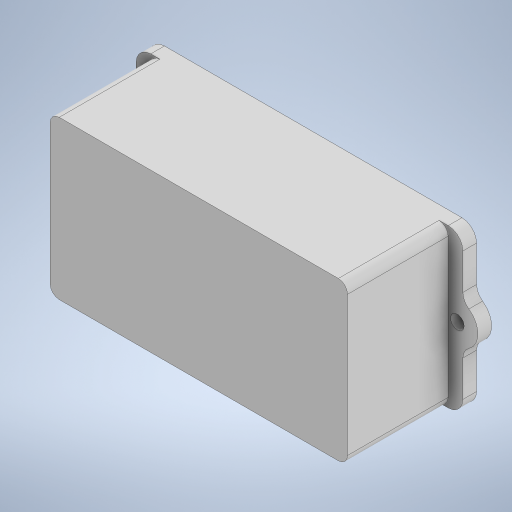
# Autodesk Inventor part: верхняя часть держателя аккумулятора
Saved by Autodesk Inventor 2023.1 (Build 271208000, 208)
## iProperties
Created: 2023-02-23
Part Number: верхняя часть держателя аккумулятора
Material: Типовые
Document SubType Name: Modeling
Designer: User
Density: 1 g/cm^3
Appearance: По умолчанию
Author: User
Autodesk Inventor part; units mm, degrees
ref_plane "YZ Plane" through (0, 0, 0) normal (1, 0, 0) x (0, 1, 0)
ref_plane "XZ Plane" through (0, 0, 0) normal (0, 1, 0) x (-1, 0, 0)
ref_plane "XY Plane" through (0, 0, 0) normal (0, 0, 1) x (1, 0, 0)
sketch "Эскиз1" plane through (0, 0, 0) normal (0, 0, 1) x (1, 0, 0)
  arc A0 (32.5, -17.25) -> (35.7, -14.05) centre (32.5, -14.05) ccw
  line L0 (35.7, -14.05) -> (35.7, -6.2137)
  arc A1 (37.02, -3.7282) -> (35.7, -6.2137) centre (38.7, -6.2137) ccw
  arc A2 (37.02, -3.7282) -> (37.02, 3.7282) centre (34.5, 0) ccw
  arc A3 (35.7, 6.2137) -> (37.02, 3.7282) centre (38.7, 6.2137) ccw
  line L1 (35.7, 6.2137) -> (35.7, 14.05)
  arc A4 (35.7, 14.05) -> (32.5, 17.25) centre (32.5, 14.05) ccw
  line L2 (32.5, 17.25) -> (-32.5, 17.25)
  arc A5 (-32.5, 17.25) -> (-35.7, 14.05) centre (-32.5, 14.05) ccw
  line L3 (-35.7, 14.05) -> (-35.7, 6.2137)
  arc A6 (-37.02, 3.7282) -> (-35.7, 6.2137) centre (-38.7, 6.2137) ccw
  arc A7 (-37.02, 3.7282) -> (-37.02, -3.7282) centre (-34.5, 0) ccw
  arc A8 (-35.7, -6.2137) -> (-37.02, -3.7282) centre (-38.7, -6.2137) ccw
  line L4 (-35.7, -6.2137) -> (-35.7, -14.05)
  arc A9 (-35.7, -14.05) -> (-32.5, -17.25) centre (-32.5, -14.05) ccw
  line L5 (-32.5, -17.25) -> (32.5, -17.25)
  line L6 (30.5, -15) -> (-30.5, -15)
  line L7 (-30.5, -15) -> (-30.5, 15)
  line L8 (-30.5, 15) -> (30.5, 15)
  line L9 (30.5, 15) -> (30.5, -15)
  circle A10 centre (-34.5, 0) radius 1.5
  circle A11 centre (34.5, 0) radius 1.5
  point P0 (0, 0)
  point P1 (-32.5, -17.25)
  point P2 (32.5, -17.25)
  point P3 (32.5, 17.25)
  point P4 (-35.7, 14.05)
  point P5 (-37.02, 3.7282)
  point P6 (-37.02, -3.7282)
  constraints: 20 end point, 20 point on circle, 12 centre point
extrude "Выдавливание1" add sketch "Эскиз1" along normal blind 3
sketch "Эскиз2" plane through (0, 0, 3) normal (0, 0, 1) x (1, 0, 0)
  line L0 (32.5, 17.25) -> (-32.5, 17.25) projected
  line L1 (-32.5, -17.25) -> (32.5, -17.25) projected
  line L2 (-32.5, 17.25) -> (32.5, 17.25)
  line L3 (32.5, 17.25) -> (32.5, -17.25)
  line L4 (32.5, -17.25) -> (-32.5, -17.25)
  line L5 (-32.5, -17.25) -> (-32.5, 17.25)
  line L6 (-30.5, 15) -> (30.5, 15) projected
  line L7 (-30.5, -15) -> (-30.5, 15) projected
  line L8 (30.5, -15) -> (-30.5, -15) projected
  line L9 (30.5, 15) -> (30.5, -15) projected
  point P0 (0, 0)
  constraints: 8 end point, 2 parallel, 1 horizontal, 1 perpendicular
extrude "Выдавливание2" add sketch "Эскиз2" along normal blind 20
fillet "Сопряжение1" radius 2 4 edges at (-32.5, -17.25, 13) (32.5, -17.25, 13) (32.5, 17.25, 13) (-32.5, 17.25, 13)
sketch "Эскиз3" plane through (0, 0, 23) normal (0, 0, 1) x (1, 0, 0)
  line L0 (30.5, 17.25) -> (-30.5, 17.25) projected
  arc A0 (-30.5, 17.25) -> (-32.5, 15.25) centre (-30.5, 15.25) ccw projected
  line L1 (-32.5, 15.25) -> (-32.5, -15.25) projected
  arc A1 (-32.5, -15.25) -> (-30.5, -17.25) centre (-30.5, -15.25) ccw projected
  line L2 (-30.5, -17.25) -> (30.5, -17.25) projected
  arc A2 (30.5, -17.25) -> (32.5, -15.25) centre (30.5, -15.25) ccw projected
  line L3 (32.5, -15.25) -> (32.5, 15.25) projected
  arc A3 (32.5, 15.25) -> (30.5, 17.25) centre (30.5, 15.25) ccw projected
  line L4 (30.5, 17.25) -> (-30.5, 17.25) projected
  line L5 (-30.5, 15) -> (30.5, 15) projected
  line L6 (30.5, 15) -> (30.5, -15) projected
  line L7 (30.5, -15) -> (-30.5, -15) projected
  line L8 (-30.5, -15) -> (-30.5, 15) projected
  point P0 (0, 0)
extrude "Выдавливание3" add sketch "Эскиз3" along normal blind 2 contours A3 L3 A2 L2 A1 L1 A0 L0 | L5 L6 L7 L8
sketch "Эскиз4" plane through (-32.5, -17.25, 0) normal (0, -1, 0) x (1, 0, 0)
  line L0 (0.3457, 22.1232) -> (67.4397, 22.1232) construction
  line L1 (67.4397, 22.1232) -> (67.4397, 17.9316) construction
  line L2 (67.4397, 17.9316) -> (0.3457, 17.9316) construction
  line L3 (0.3457, 17.9316) -> (0.3457, 22.1232) construction
  line L4 (7.2699, 17.9367) -> (6.3706, 17.9367)
  spline S0 degree 2 poles (6.3706, 17.9367) (6.0759, 17.9367) (6.0759, 18.2364) knots 0 0 0 1 1 1
  spline S1 degree 2 poles (6.0759, 18.2364) (6.0759, 18.5362) (6.3706, 18.5362) knots 0 0 0 1 1 1
  line L5 (6.3706, 18.5362) -> (7.2699, 18.5362)
  line L6 (7.2699, 18.5362) -> (7.2699, 19.1357)
  spline S2 degree 2 poles (7.2699, 19.1357) (7.2699, 19.3805) (6.9152, 19.7302) (6.6704, 19.7302) knots 0 0 0 1 2 2 2
  line L7 (6.6704, 19.7302) -> (5.1766, 19.7302)
  spline S3 degree 2 poles (5.1766, 19.7302) (4.8769, 19.7302) (4.8769, 20.0299) knots 0 0 0 1 1 1
  spline S4 degree 2 poles (4.8769, 20.0299) (4.8769, 20.3297) (5.1766, 20.3297) knots 0 0 0 1 1 1
  line L8 (5.1766, 20.3297) -> (6.6704, 20.3297)
  spline S5 degree 2 poles (6.6704, 20.3297) (7.17, 20.3297) (7.8694, 19.6303) (7.8694, 19.1357) knots 0 0 0 1 2 2 2
  line L9 (7.8694, 19.1357) -> (7.8694, 17.3372)
  spline S6 degree 2 poles (7.8694, 17.3372) (7.8694, 16.8426) (7.17, 16.1432) (6.6704, 16.1432) knots 0 0 0 1 2 2 2
  line L10 (6.6704, 16.1432) -> (5.1766, 16.1432)
  spline S7 degree 2 poles (5.1766, 16.1432) (4.8769, 16.1432) (4.8769, 16.4429) knots 0 0 0 1 1 1
  spline S8 degree 2 poles (4.8769, 16.4429) (4.8769, 16.7427) (5.1766, 16.7427) knots 0 0 0 1 1 1
  line L11 (5.1766, 16.7427) -> (6.6704, 16.7427)
  spline S9 degree 2 poles (6.6704, 16.7427) (6.9152, 16.7427) (7.2699, 17.0974) (7.2699, 17.3422) knots 0 0 0 1 2 2 2
  line L12 (7.2699, 17.3422) -> (7.2699, 17.9367)
  line L13 (10.8619, 19.7302) -> (9.6679, 19.7302)
  line L14 (9.6679, 19.7302) -> (9.6679, 16.4429)
  spline S10 degree 2 poles (9.6679, 16.4429) (9.6679, 16.1432) (9.3681, 16.1432) knots 0 0 0 1 1 1
  spline S11 degree 2 poles (9.3681, 16.1432) (9.0684, 16.1432) (9.0684, 16.4429) knots 0 0 0 1 1 1
  line L15 (9.0684, 16.4429) -> (9.0684, 20.0299)
  spline S12 degree 2 poles (9.0684, 20.0299) (9.0684, 20.3297) (9.3681, 20.3297) knots 0 0 0 1 1 1
  line L16 (9.3681, 20.3297) -> (12.0609, 20.3297)
  spline S13 degree 2 poles (12.0609, 20.3297) (12.5555, 20.3297) (13.2549, 19.6303) (13.2549, 19.1357) knots 0 0 0 1 2 2 2
  line L17 (13.2549, 19.1357) -> (13.2549, 16.4429)
  spline S14 degree 2 poles (13.2549, 16.4429) (13.2549, 16.1432) (12.9551, 16.1432) knots 0 0 0 1 1 1
  spline S15 degree 2 poles (12.9551, 16.1432) (12.6554, 16.1432) (12.6554, 16.4429) knots 0 0 0 1 1 1
  line L18 (12.6554, 16.4429) -> (12.6554, 19.1307)
  spline S16 degree 2 poles (12.6554, 19.1307) (12.6554, 19.3755) (12.3057, 19.7302) (12.0609, 19.7302) knots 0 0 0 1 2 2 2
  line L19 (12.0609, 19.7302) -> (11.4614, 19.7302)
  line L20 (11.4614, 19.7302) -> (11.4614, 16.4429)
  spline S17 degree 2 poles (11.4614, 16.4429) (11.4614, 16.1432) (11.1616, 16.1432) knots 0 0 0 1 1 1
  spline S18 degree 2 poles (11.1616, 16.1432) (10.8619, 16.1432) (10.8619, 16.4429) knots 0 0 0 1 1 1
  line L21 (10.8619, 16.4429) -> (10.8619, 19.7302)
  spline S19 degree 2 poles (17.4414, 17.4571) (17.4414, 16.9075) (16.672, 16.1432) (16.1275, 16.1432) knots 0 0 0 1 2 2 2
  line L22 (16.1275, 16.1432) -> (15.7678, 16.1432)
  spline S20 degree 2 poles (15.7678, 16.1432) (15.2282, 16.1432) (14.4539, 16.9125) (14.4539, 17.4571) knots 0 0 0 1 2 2 2
  line L23 (14.4539, 17.4571) -> (14.4539, 19.0158)
  spline S21 degree 2 poles (14.4539, 19.0158) (14.4539, 19.5603) (15.2282, 20.3297) (15.7678, 20.3297) knots 0 0 0 1 2 2 2
  line L24 (15.7678, 20.3297) -> (16.1275, 20.3297)
  spline S22 degree 2 poles (16.1275, 20.3297) (16.672, 20.3297) (17.4414, 19.5603) (17.4414, 19.0158) knots 0 0 0 1 2 2 2
  line L25 (17.4414, 19.0158) -> (17.4414, 17.4571)
  line L26 (16.8419, 17.4621) -> (16.8419, 19.0108)
  spline S23 degree 2 poles (16.8419, 19.0108) (16.8419, 19.3055) (16.4172, 19.7302) (16.1275, 19.7302) knots 0 0 0 1 2 2 2
  line L27 (16.1275, 19.7302) -> (15.7678, 19.7302)
  spline S24 degree 2 poles (15.7678, 19.7302) (15.473, 19.7302) (15.0534, 19.3055) (15.0534, 19.0108) knots 0 0 0 1 2 2 2
  line L28 (15.0534, 19.0108) -> (15.0534, 17.4621)
  spline S25 degree 2 poles (15.0534, 17.4621) (15.0534, 17.1623) (15.473, 16.7427) (15.7678, 16.7427) knots 0 0 0 1 2 2 2
  line L29 (15.7678, 16.7427) -> (16.1275, 16.7427)
  spline S26 degree 2 poles (16.1275, 16.7427) (16.4172, 16.7427) (16.8419, 17.1623) (16.8419, 17.4621) knots 0 0 0 1 2 2 2
  spline S27 degree 2 poles (21.6329, 16.4429) (21.6329, 16.1432) (21.3332, 16.1432) knots 0 0 0 1 1 1
  line L30 (21.3332, 16.1432) -> (19.8394, 16.1432)
  spline S28 degree 2 poles (19.8394, 16.1432) (19.3448, 16.1432) (18.6404, 16.8426) (18.6404, 17.3422) knots 0 0 0 1 2 2 2
  line L31 (18.6404, 17.3422) -> (18.6404, 20.0349)
  spline S29 degree 2 poles (18.6404, 20.0349) (18.6404, 20.3297) (18.9401, 20.3297) knots 0 0 0 1 1 1
  spline S30 degree 2 poles (18.9401, 20.3297) (19.2399, 20.3297) (19.2399, 20.0349) knots 0 0 0 1 1 1
  line L32 (19.2399, 20.0349) -> (19.2399, 17.3422)
  spline S31 degree 2 poles (19.2399, 17.3422) (19.2399, 17.0974) (19.5946, 16.7427) (19.8394, 16.7427) knots 0 0 0 1 2 2 2
  line L33 (19.8394, 16.7427) -> (21.0334, 16.7427)
  line L34 (21.0334, 16.7427) -> (21.0334, 20.0349)
  spline S32 degree 2 poles (21.0334, 20.0349) (21.0334, 20.3297) (21.3332, 20.3297) knots 0 0 0 1 1 1
  spline S33 degree 2 poles (21.3332, 20.3297) (21.6329, 20.3297) (21.6329, 20.0349) knots 0 0 0 1 1 1
  line L35 (21.6329, 20.0349) -> (21.6329, 16.4429)
  line L36 (20.7337, 21.5237) -> (19.5396, 21.5237)
  spline S34 degree 2 poles (19.5396, 21.5237) (19.2399, 21.5237) (19.2399, 21.8234) knots 0 0 0 1 1 1
  spline S35 degree 2 poles (19.2399, 21.8234) (19.2399, 22.1232) (19.5396, 22.1232) knots 0 0 0 1 1 1
  line L37 (19.5396, 22.1232) -> (20.7337, 22.1232)
  spline S36 degree 2 poles (20.7337, 22.1232) (21.0334, 22.1232) (21.0334, 21.8234) knots 0 0 0 1 1 1
  spline S37 degree 2 poles (21.0334, 21.8234) (21.0334, 21.5237) (20.7337, 21.5237) knots 0 0 0 1 1 1
  line L38 (28.5122, 16.1432) -> (27.6179, 16.1432)
  spline S38 degree 2 poles (27.6179, 16.1432) (27.1283, 16.1432) (26.4189, 16.8426) (26.4189, 17.3372) knots 0 0 0 1 2 2 2
  line L39 (26.4189, 17.3372) -> (26.4189, 19.1357)
  spline S39 degree 2 poles (26.4189, 19.1357) (26.4189, 19.6303) (27.1283, 20.3297) (27.6179, 20.3297) knots 0 0 0 1 2 2 2
  line L40 (27.6179, 20.3297) -> (28.5122, 20.3297)
  spline S40 degree 2 poles (28.5122, 20.3297) (28.8119, 20.3297) (28.8119, 20.0299) knots 0 0 0 1 1 1
  spline S41 degree 2 poles (28.8119, 20.0299) (28.8119, 19.7302) (28.5122, 19.7302) knots 0 0 0 1 1 1
  line L41 (28.5122, 19.7302) -> (27.6179, 19.7302)
  spline S42 degree 2 poles (27.6179, 19.7302) (27.3731, 19.7302) (27.0184, 19.3755) (27.0184, 19.1307) knots 0 0 0 1 2 2 2
  line L42 (27.0184, 19.1307) -> (27.0184, 17.3422)
  spline S43 degree 2 poles (27.0184, 17.3422) (27.0184, 17.0974) (27.3731, 16.7427) (27.6179, 16.7427) knots 0 0 0 1 2 2 2
  line L43 (27.6179, 16.7427) -> (28.5122, 16.7427)
  spline S44 degree 2 poles (28.5122, 16.7427) (28.8119, 16.7427) (28.8119, 16.4429) knots 0 0 0 1 1 1
  spline S45 degree 2 poles (28.8119, 16.4429) (28.8119, 16.1432) (28.5122, 16.1432) knots 0 0 0 1 1 1
  line L44 (31.7994, 19.7302) -> (30.6054, 19.7302)
  line L45 (30.6054, 19.7302) -> (30.6054, 16.4429)
  spline S46 degree 2 poles (30.6054, 16.4429) (30.6054, 16.1432) (30.3057, 16.1432) knots 0 0 0 1 1 1
  spline S47 degree 2 poles (30.3057, 16.1432) (30.0059, 16.1432) (30.0059, 16.4429) knots 0 0 0 1 1 1
  line L46 (30.0059, 16.4429) -> (30.0059, 20.0299)
  spline S48 degree 2 poles (30.0059, 20.0299) (30.0059, 20.3297) (30.3057, 20.3297) knots 0 0 0 1 1 1
  line L47 (30.3057, 20.3297) -> (32.9984, 20.3297)
  spline S49 degree 2 poles (32.9984, 20.3297) (33.493, 20.3297) (34.1924, 19.6303) (34.1924, 19.1357) knots 0 0 0 1 2 2 2
  line L48 (34.1924, 19.1357) -> (34.1924, 16.4429)
  spline S50 degree 2 poles (34.1924, 16.4429) (34.1924, 16.1432) (33.8927, 16.1432) knots 0 0 0 1 1 1
  spline S51 degree 2 poles (33.8927, 16.1432) (33.5929, 16.1432) (33.5929, 16.4429) knots 0 0 0 1 1 1
  line L49 (33.5929, 16.4429) -> (33.5929, 19.1307)
  spline S52 degree 2 poles (33.5929, 19.1307) (33.5929, 19.3755) (33.2432, 19.7302) (32.9984, 19.7302) knots 0 0 0 1 2 2 2
  line L50 (32.9984, 19.7302) -> (32.3989, 19.7302)
  line L51 (32.3989, 19.7302) -> (32.3989, 16.4429)
  spline S53 degree 2 poles (32.3989, 16.4429) (32.3989, 16.1432) (32.0992, 16.1432) knots 0 0 0 1 1 1
  spline S54 degree 2 poles (32.0992, 16.1432) (31.7994, 16.1432) (31.7994, 16.4429) knots 0 0 0 1 1 1
  line L52 (31.7994, 16.4429) -> (31.7994, 19.7302)
  spline S55 degree 2 poles (38.3789, 17.4571) (38.3789, 16.9075) (37.6096, 16.1432) (37.065, 16.1432) knots 0 0 0 1 2 2 2
  line L53 (37.065, 16.1432) -> (36.7053, 16.1432)
  spline S56 degree 2 poles (36.7053, 16.1432) (36.1658, 16.1432) (35.3914, 16.9125) (35.3914, 17.4571) knots 0 0 0 1 2 2 2
  line L54 (35.3914, 17.4571) -> (35.3914, 19.0158)
  spline S57 degree 2 poles (35.3914, 19.0158) (35.3914, 19.5603) (36.1658, 20.3297) (36.7053, 20.3297) knots 0 0 0 1 2 2 2
  line L55 (36.7053, 20.3297) -> (37.065, 20.3297)
  spline S58 degree 2 poles (37.065, 20.3297) (37.6096, 20.3297) (38.3789, 19.5603) (38.3789, 19.0158) knots 0 0 0 1 2 2 2
  line L56 (38.3789, 19.0158) -> (38.3789, 17.4571)
  line L57 (37.7794, 17.4621) -> (37.7794, 19.0108)
  spline S59 degree 2 poles (37.7794, 19.0108) (37.7794, 19.3055) (37.3548, 19.7302) (37.065, 19.7302) knots 0 0 0 1 2 2 2
  line L58 (37.065, 19.7302) -> (36.7053, 19.7302)
  spline S60 degree 2 poles (36.7053, 19.7302) (36.4106, 19.7302) (35.9909, 19.3055) (35.9909, 19.0108) knots 0 0 0 1 2 2 2
  line L59 (35.9909, 19.0108) -> (35.9909, 17.4621)
  spline S61 degree 2 poles (35.9909, 17.4621) (35.9909, 17.1623) (36.4106, 16.7427) (36.7053, 16.7427) knots 0 0 0 1 2 2 2
  line L60 (36.7053, 16.7427) -> (37.065, 16.7427)
  spline S62 degree 2 poles (37.065, 16.7427) (37.3548, 16.7427) (37.7794, 17.1623) (37.7794, 17.4621) knots 0 0 0 1 2 2 2
  line L61 (40.1774, 16.1432) -> (40.1774, 14.6494)
  spline S63 degree 2 poles (40.1774, 14.6494) (40.1774, 14.3497) (39.8777, 14.3497) knots 0 0 0 1 1 1
  spline S64 degree 2 poles (39.8777, 14.3497) (39.5779, 14.3497) (39.5779, 14.6494) knots 0 0 0 1 1 1
  line L62 (39.5779, 14.6494) -> (39.5779, 20.0299)
  spline S65 degree 2 poles (39.5779, 20.0299) (39.5779, 20.3297) (39.8777, 20.3297) knots 0 0 0 1 1 1
  line L63 (39.8777, 20.3297) -> (41.3715, 20.3297)
  spline S66 degree 2 poles (41.3715, 20.3297) (41.866, 20.3297) (42.5655, 19.6303) (42.5655, 19.1357) knots 0 0 0 1 2 2 2
  line L64 (42.5655, 19.1357) -> (42.5655, 17.3372)
  spline S67 degree 2 poles (42.5655, 17.3372) (42.5655, 16.8426) (41.866, 16.1432) (41.3715, 16.1432) knots 0 0 0 1 2 2 2
  line L65 (41.3715, 16.1432) -> (40.1774, 16.1432)
  line L66 (40.1774, 16.7427) -> (41.3715, 16.7427)
  spline S68 degree 2 poles (41.3715, 16.7427) (41.6162, 16.7427) (41.966, 17.0974) (41.966, 17.3422) knots 0 0 0 1 2 2 2
  line L67 (41.966, 17.3422) -> (41.966, 19.1307)
  spline S69 degree 2 poles (41.966, 19.1307) (41.966, 19.3755) (41.6162, 19.7302) (41.3715, 19.7302) knots 0 0 0 1 2 2 2
  line L68 (41.3715, 19.7302) -> (40.1774, 19.7302)
  line L69 (40.1774, 19.7302) -> (40.1774, 16.7427)
  spline S70 degree 2 poles (46.752, 17.4571) (46.752, 16.9075) (45.9826, 16.1432) (45.4381, 16.1432) knots 0 0 0 1 2 2 2
  line L70 (45.4381, 16.1432) -> (45.0784, 16.1432)
  spline S71 degree 2 poles (45.0784, 16.1432) (44.5388, 16.1432) (43.7645, 16.9125) (43.7645, 17.4571) knots 0 0 0 1 2 2 2
  line L71 (43.7645, 17.4571) -> (43.7645, 19.0158)
  spline S72 degree 2 poles (43.7645, 19.0158) (43.7645, 19.5603) (44.5388, 20.3297) (45.0784, 20.3297) knots 0 0 0 1 2 2 2
  line L72 (45.0784, 20.3297) -> (45.4381, 20.3297)
  spline S73 degree 2 poles (45.4381, 20.3297) (45.9826, 20.3297) (46.752, 19.5603) (46.752, 19.0158) knots 0 0 0 1 2 2 2
  line L73 (46.752, 19.0158) -> (46.752, 17.4571)
  line L74 (46.1525, 17.4621) -> (46.1525, 19.0108)
  spline S74 degree 2 poles (46.1525, 19.0108) (46.1525, 19.3055) (45.7278, 19.7302) (45.4381, 19.7302) knots 0 0 0 1 2 2 2
  line L75 (45.4381, 19.7302) -> (45.0784, 19.7302)
  spline S75 degree 2 poles (45.0784, 19.7302) (44.7836, 19.7302) (44.364, 19.3055) (44.364, 19.0108) knots 0 0 0 1 2 2 2
  line L76 (44.364, 19.0108) -> (44.364, 17.4621)
  spline S76 degree 2 poles (44.364, 17.4621) (44.364, 17.1623) (44.7836, 16.7427) (45.0784, 16.7427) knots 0 0 0 1 2 2 2
  line L77 (45.0784, 16.7427) -> (45.4381, 16.7427)
  spline S77 degree 2 poles (45.4381, 16.7427) (45.7278, 16.7427) (46.1525, 17.1623) (46.1525, 17.4621) knots 0 0 0 1 2 2 2
  line L78 (50.339, 18.5362) -> (50.339, 20.0299)
  spline S78 degree 2 poles (50.339, 20.0299) (50.339, 20.3297) (50.6387, 20.3297) knots 0 0 0 1 1 1
  spline S79 degree 2 poles (50.6387, 20.3297) (50.9385, 20.3297) (50.9385, 20.0299) knots 0 0 0 1 1 1
  line L79 (50.9385, 20.0299) -> (50.9385, 16.4429)
  spline S80 degree 2 poles (50.9385, 16.4429) (50.9385, 16.1432) (50.6387, 16.1432) knots 0 0 0 1 1 1
  spline S81 degree 2 poles (50.6387, 16.1432) (50.339, 16.1432) (50.339, 16.4429) knots 0 0 0 1 1 1
  line L80 (50.339, 16.4429) -> (50.339, 17.9367)
  line L81 (50.339, 17.9367) -> (48.5505, 17.9367)
  line L82 (48.5505, 17.9367) -> (48.5505, 16.4429)
  spline S82 degree 2 poles (48.5505, 16.4429) (48.5505, 16.1432) (48.2507, 16.1432) knots 0 0 0 1 1 1
  spline S83 degree 2 poles (48.2507, 16.1432) (47.951, 16.1432) (47.951, 16.4429) knots 0 0 0 1 1 1
  line L83 (47.951, 16.4429) -> (47.951, 20.0299)
  spline S84 degree 2 poles (47.951, 20.0299) (47.951, 20.3297) (48.2507, 20.3297) knots 0 0 0 1 1 1
  spline S85 degree 2 poles (48.2507, 20.3297) (48.5505, 20.3297) (48.5505, 20.0299) knots 0 0 0 1 1 1
  line L84 (48.5505, 20.0299) -> (48.5505, 18.5362)
  line L85 (48.5505, 18.5362) -> (50.339, 18.5362)
  spline S86 degree 2 poles (55.125, 17.4571) (55.125, 16.9075) (54.3556, 16.1432) (53.8111, 16.1432) knots 0 0 0 1 2 2 2
  line L86 (53.8111, 16.1432) -> (53.4514, 16.1432)
  spline S87 degree 2 poles (53.4514, 16.1432) (52.9118, 16.1432) (52.1375, 16.9125) (52.1375, 17.4571) knots 0 0 0 1 2 2 2
  line L87 (52.1375, 17.4571) -> (52.1375, 19.0158)
  spline S88 degree 2 poles (52.1375, 19.0158) (52.1375, 19.5603) (52.9118, 20.3297) (53.4514, 20.3297) knots 0 0 0 1 2 2 2
  line L88 (53.4514, 20.3297) -> (53.8111, 20.3297)
  spline S89 degree 2 poles (53.8111, 20.3297) (54.3556, 20.3297) (55.125, 19.5603) (55.125, 19.0158) knots 0 0 0 1 2 2 2
  line L89 (55.125, 19.0158) -> (55.125, 17.4571)
  line L90 (54.5255, 17.4621) -> (54.5255, 19.0108)
  spline S90 degree 2 poles (54.5255, 19.0108) (54.5255, 19.3055) (54.1008, 19.7302) (53.8111, 19.7302) knots 0 0 0 1 2 2 2
  line L91 (53.8111, 19.7302) -> (53.4514, 19.7302)
  spline S91 degree 2 poles (53.4514, 19.7302) (53.1566, 19.7302) (52.737, 19.3055) (52.737, 19.0108) knots 0 0 0 1 2 2 2
  line L92 (52.737, 19.0108) -> (52.737, 17.4621)
  spline S92 degree 2 poles (52.737, 17.4621) (52.737, 17.1623) (53.1566, 16.7427) (53.4514, 16.7427) knots 0 0 0 1 2 2 2
  line L93 (53.4514, 16.7427) -> (53.8111, 16.7427)
  spline S93 degree 2 poles (53.8111, 16.7427) (54.1008, 16.7427) (54.5255, 17.1623) (54.5255, 17.4621) knots 0 0 0 1 2 2 2
  spline S94 degree 2 poles (59.3165, 16.4429) (59.3165, 16.1432) (59.0168, 16.1432) knots 0 0 0 1 1 1
  line L94 (59.0168, 16.1432) -> (57.523, 16.1432)
  spline S95 degree 2 poles (57.523, 16.1432) (57.0284, 16.1432) (56.324, 16.8426) (56.324, 17.3422) knots 0 0 0 1 2 2 2
  line L95 (56.324, 17.3422) -> (56.324, 20.0349)
  spline S96 degree 2 poles (56.324, 20.0349) (56.324, 20.3297) (56.6237, 20.3297) knots 0 0 0 1 1 1
  spline S97 degree 2 poles (56.6237, 20.3297) (56.9235, 20.3297) (56.9235, 20.0349) knots 0 0 0 1 1 1
  line L96 (56.9235, 20.0349) -> (56.9235, 17.3422)
  spline S98 degree 2 poles (56.9235, 17.3422) (56.9235, 17.0974) (57.2782, 16.7427) (57.523, 16.7427) knots 0 0 0 1 2 2 2
  line L97 (57.523, 16.7427) -> (58.717, 16.7427)
  line L98 (58.717, 16.7427) -> (58.717, 20.0349)
  spline S99 degree 2 poles (58.717, 20.0349) (58.717, 20.3297) (59.0168, 20.3297) knots 0 0 0 1 1 1
  spline S100 degree 2 poles (59.0168, 20.3297) (59.3165, 20.3297) (59.3165, 20.0349) knots 0 0 0 1 1 1
  line L99 (59.3165, 20.0349) -> (59.3165, 16.4429)
  line L100 (58.4172, 21.5237) -> (57.2232, 21.5237)
  spline S101 degree 2 poles (57.2232, 21.5237) (56.9235, 21.5237) (56.9235, 21.8234) knots 0 0 0 1 1 1
  spline S102 degree 2 poles (56.9235, 21.8234) (56.9235, 22.1232) (57.2232, 22.1232) knots 0 0 0 1 1 1
  line L101 (57.2232, 22.1232) -> (58.4172, 22.1232)
  spline S103 degree 2 poles (58.4172, 22.1232) (58.717, 22.1232) (58.717, 21.8234) knots 0 0 0 1 1 1
  spline S104 degree 2 poles (58.717, 21.8234) (58.717, 21.5237) (58.4172, 21.5237) knots 0 0 0 1 1 1
  line L102 (22.8269, 8.2642) -> (22.8269, 9.7579)
  spline S105 degree 2 poles (22.8269, 9.7579) (22.8269, 10.0577) (23.1267, 10.0577) knots 0 0 0 1 1 1
  spline S106 degree 2 poles (23.1267, 10.0577) (23.4264, 10.0577) (23.4264, 9.7579) knots 0 0 0 1 1 1
  line L103 (23.4264, 9.7579) -> (23.4264, 6.1709)
  spline S107 degree 2 poles (23.4264, 6.1709) (23.4264, 5.8712) (23.1267, 5.8712) knots 0 0 0 1 1 1
  spline S108 degree 2 poles (23.1267, 5.8712) (22.8269, 5.8712) (22.8269, 6.1709) knots 0 0 0 1 1 1
  line L104 (22.8269, 6.1709) -> (22.8269, 7.6647)
  line L105 (22.8269, 7.6647) -> (21.0384, 7.6647)
  line L106 (21.0384, 7.6647) -> (21.0384, 6.1709)
  spline S109 degree 2 poles (21.0384, 6.1709) (21.0384, 5.8712) (20.7386, 5.8712) knots 0 0 0 1 1 1
  spline S110 degree 2 poles (20.7386, 5.8712) (20.4389, 5.8712) (20.4389, 6.1709) knots 0 0 0 1 1 1
  line L107 (20.4389, 6.1709) -> (20.4389, 9.7579)
  spline S111 degree 2 poles (20.4389, 9.7579) (20.4389, 10.0577) (20.7386, 10.0577) knots 0 0 0 1 1 1
  spline S112 degree 2 poles (20.7386, 10.0577) (21.0384, 10.0577) (21.0384, 9.7579) knots 0 0 0 1 1 1
  line L108 (21.0384, 9.7579) -> (21.0384, 8.2642)
  line L109 (21.0384, 8.2642) -> (22.8269, 8.2642)
  spline S113 degree 2 poles (27.3082, 6.2659) (26.9485, 5.8712) (26.4189, 5.8712) knots 0 0 0 1 1 1
  line L110 (26.4189, 5.8712) -> (25.8194, 5.8712)
  spline S114 degree 2 poles (25.8194, 5.8712) (25.3298, 5.8712) (24.6254, 6.5706) (24.6254, 7.0652) knots 0 0 0 1 2 2 2
  line L111 (24.6254, 7.0652) -> (24.6254, 8.8637)
  spline S115 degree 2 poles (24.6254, 8.8637) (24.6254, 9.3583) (25.3298, 10.0577) (25.8194, 10.0577) knots 0 0 0 1 2 2 2
  line L112 (25.8194, 10.0577) -> (27.3132, 10.0577)
  spline S116 degree 2 poles (27.3132, 10.0577) (27.6129, 10.0577) (27.6129, 9.7579) knots 0 0 0 1 1 1
  line L113 (27.6129, 9.7579) -> (27.6129, 7.0752)
  spline S117 degree 2 poles (27.6129, 7.0752) (27.6129, 6.6256) (28.0326, 6.4457) knots 0 0 0 1 1 1
  spline S118 degree 2 poles (28.0326, 6.4457) (28.2174, 6.3708) (28.2174, 6.1809) knots 0 0 0 1 1 1
  spline S119 degree 2 poles (28.2174, 6.1809) (28.2174, 6.056) (28.0476, 5.8662) (27.9227, 5.8662) knots 0 0 0 1 2 2 2
  spline S120 degree 2 poles (27.9227, 5.8662) (27.8577, 5.8662) (27.7928, 5.8962) knots 0 0 0 1 1 1
  spline S121 degree 2 poles (27.7928, 5.8962) (27.493, 6.0261) (27.3082, 6.2659) knots 0 0 0 1 1 1
  line L114 (27.0134, 7.0702) -> (27.0134, 9.4582)
  line L115 (27.0134, 9.4582) -> (25.8194, 9.4582)
  spline S122 degree 2 poles (25.8194, 9.4582) (25.5746, 9.4582) (25.2249, 9.1035) (25.2249, 8.8587) knots 0 0 0 1 2 2 2
  line L116 (25.2249, 8.8587) -> (25.2249, 7.0702)
  spline S123 degree 2 poles (25.2249, 7.0702) (25.2249, 6.8254) (25.5746, 6.4707) (25.8194, 6.4707) knots 0 0 0 1 2 2 2
  line L117 (25.8194, 6.4707) -> (26.4189, 6.4707)
  spline S124 degree 2 poles (26.4189, 6.4707) (26.6637, 6.4707) (27.0134, 6.8254) (27.0134, 7.0702) knots 0 0 0 1 2 2 2
  line L118 (34.4922, 5.8712) -> (33.5979, 5.8712)
  spline S125 degree 2 poles (33.5979, 5.8712) (33.1083, 5.8712) (32.3989, 6.5706) (32.3989, 7.0652) knots 0 0 0 1 2 2 2
  line L119 (32.3989, 7.0652) -> (32.3989, 8.8637)
  spline S126 degree 2 poles (32.3989, 8.8637) (32.3989, 9.3583) (33.1083, 10.0577) (33.5979, 10.0577) knots 0 0 0 1 2 2 2
  line L120 (33.5979, 10.0577) -> (34.4922, 10.0577)
  spline S127 degree 2 poles (34.4922, 10.0577) (34.7919, 10.0577) (34.7919, 9.7579) knots 0 0 0 1 1 1
  spline S128 degree 2 poles (34.7919, 9.7579) (34.7919, 9.4582) (34.4922, 9.4582) knots 0 0 0 1 1 1
  line L121 (34.4922, 9.4582) -> (33.5979, 9.4582)
  spline S129 degree 2 poles (33.5979, 9.4582) (33.3531, 9.4582) (32.9984, 9.1035) (32.9984, 8.8587) knots 0 0 0 1 2 2 2
  line L122 (32.9984, 8.8587) -> (32.9984, 7.0702)
  spline S130 degree 2 poles (32.9984, 7.0702) (32.9984, 6.8254) (33.3531, 6.4707) (33.5979, 6.4707) knots 0 0 0 1 2 2 2
  line L123 (33.5979, 6.4707) -> (34.4922, 6.4707)
  spline S131 degree 2 poles (34.4922, 6.4707) (34.7919, 6.4707) (34.7919, 6.1709) knots 0 0 0 1 1 1
  spline S132 degree 2 poles (34.7919, 6.1709) (34.7919, 5.8712) (34.4922, 5.8712) knots 0 0 0 1 1 1
  line L124 (36.5854, 7.6647) -> (36.5854, 7.0702)
  spline S133 degree 2 poles (36.5854, 7.0702) (36.5854, 6.8254) (36.9401, 6.4707) (37.1849, 6.4707) knots 0 0 0 1 2 2 2
  line L125 (37.1849, 6.4707) -> (38.6737, 6.4707)
  spline S134 degree 2 poles (38.6737, 6.4707) (38.9735, 6.4707) (38.9735, 6.1709) knots 0 0 0 1 1 1
  spline S135 degree 2 poles (38.9735, 6.1709) (38.9735, 5.8712) (38.6737, 5.8712) knots 0 0 0 1 1 1
  line L126 (38.6737, 5.8712) -> (37.1799, 5.8712)
  spline S136 degree 2 poles (37.1799, 5.8712) (36.6854, 5.8712) (35.9859, 6.5706) (35.9859, 7.0652) knots 0 0 0 1 2 2 2
  line L127 (35.9859, 7.0652) -> (35.9859, 8.8637)
  spline S137 degree 2 poles (35.9859, 8.8637) (35.9859, 9.3583) (36.6854, 10.0577) (37.1799, 10.0577) knots 0 0 0 1 2 2 2
  line L128 (37.1799, 10.0577) -> (37.7794, 10.0577)
  spline S138 degree 2 poles (37.7794, 10.0577) (38.274, 10.0577) (38.9735, 9.3583) (38.9735, 8.8637) knots 0 0 0 1 2 2 2
  line L129 (38.9735, 8.8637) -> (38.9735, 7.9644)
  spline S139 degree 2 poles (38.9735, 7.9644) (38.9735, 7.6647) (38.6737, 7.6647) knots 0 0 0 1 1 1
  line L130 (38.6737, 7.6647) -> (36.5854, 7.6647)
  line L131 (36.5854, 8.2642) -> (38.374, 8.2642)
  line L132 (38.374, 8.2642) -> (38.374, 8.8637)
  spline S140 degree 2 poles (38.374, 8.8637) (38.374, 9.1085) (38.0242, 9.4582) (37.7794, 9.4582) knots 0 0 0 1 2 2 2
  line L133 (37.7794, 9.4582) -> (37.1799, 9.4582)
  spline S141 degree 2 poles (37.1799, 9.4582) (36.9352, 9.4582) (36.5854, 9.1085) (36.5854, 8.8637) knots 0 0 0 1 2 2 2
  line L134 (36.5854, 8.8637) -> (36.5854, 8.2642)
  line L135 (41.6013, 10.0577) -> (40.2624, 11.3366)
  spline S142 degree 2 poles (40.2624, 11.3366) (40.1525, 11.4465) (40.1525, 11.5814) knots 0 0 0 1 1 1
  spline S143 degree 2 poles (40.1525, 11.5814) (40.1525, 11.8512) (40.4672, 11.8512) knots 0 0 0 1 1 1
  line L136 (40.4672, 11.8512) -> (42.8602, 11.8512)
  spline S144 degree 2 poles (42.8602, 11.8512) (43.16, 11.8512) (43.16, 11.5515) knots 0 0 0 1 1 1
  spline S145 degree 2 poles (43.16, 11.5515) (43.16, 11.2517) (42.8602, 11.2517) knots 0 0 0 1 1 1
  line L137 (42.8602, 11.2517) -> (41.2166, 11.2517)
  line L138 (41.2166, 11.2517) -> (42.8003, 9.738)
  spline S146 degree 2 poles (42.8003, 9.738) (42.8502, 9.698) (42.8752, 9.643) knots 0 0 0 1 1 1
  spline S147 degree 2 poles (42.8752, 9.643) (43.16, 9.3083) (43.16, 8.8587) knots 0 0 0 1 1 1
  line L139 (43.16, 8.8587) -> (43.16, 7.0652)
  spline S148 degree 2 poles (43.16, 7.0652) (43.16, 6.5706) (42.4605, 5.8712) (41.966, 5.8712) knots 0 0 0 1 2 2 2
  line L140 (41.966, 5.8712) -> (41.3665, 5.8712)
  spline S149 degree 2 poles (41.3665, 5.8712) (40.8769, 5.8712) (40.1725, 6.5706) (40.1725, 7.0652) knots 0 0 0 1 2 2 2
  line L141 (40.1725, 7.0652) -> (40.1725, 8.8637)
  spline S150 degree 2 poles (40.1725, 8.8637) (40.1725, 9.3583) (40.8769, 10.0577) (41.3665, 10.0577) knots 0 0 0 1 2 2 2
  line L142 (41.3665, 10.0577) -> (41.6013, 10.0577)
  line L143 (42.5605, 7.0702) -> (42.5605, 8.8587)
  spline S151 degree 2 poles (42.5605, 8.8587) (42.5605, 9.1035) (42.2108, 9.4582) (41.966, 9.4582) knots 0 0 0 1 2 2 2
  line L144 (41.966, 9.4582) -> (41.3665, 9.4582)
  spline S152 degree 2 poles (41.3665, 9.4582) (41.1217, 9.4582) (40.772, 9.1035) (40.772, 8.8587) knots 0 0 0 1 2 2 2
  line L145 (40.772, 8.8587) -> (40.772, 7.0702)
  spline S153 degree 2 poles (40.772, 7.0702) (40.772, 6.8254) (41.1217, 6.4707) (41.3665, 6.4707) knots 0 0 0 1 2 2 2
  line L146 (41.3665, 6.4707) -> (41.966, 6.4707)
  spline S154 degree 2 poles (41.966, 6.4707) (42.2108, 6.4707) (42.5605, 6.8254) (42.5605, 7.0702) knots 0 0 0 1 2 2 2
  line L147 (46.0126, 7.6647) -> (44.9085, 6.0061)
  spline S155 degree 2 poles (44.9085, 6.0061) (44.8186, 5.8662) (44.6687, 5.8662) knots 0 0 0 1 1 1
  spline S156 degree 2 poles (44.6687, 5.8662) (44.5438, 5.8662) (44.354, 6.046) (44.354, 6.1659) knots 0 0 0 1 2 2 2
  spline S157 degree 2 poles (44.354, 6.1659) (44.354, 6.2559) (44.4089, 6.3358) knots 0 0 0 1 1 1
  line L148 (44.4089, 6.3358) -> (45.3082, 7.6847)
  spline S158 degree 2 poles (45.3082, 7.6847) (44.8585, 7.7596) (44.5938, 8.1143) knots 0 0 0 1 1 1
  spline S159 degree 2 poles (44.5938, 8.1143) (44.359, 8.4341) (44.359, 8.8637) knots 0 0 0 1 1 1
  spline S160 degree 2 poles (44.359, 8.8637) (44.359, 9.3483) (44.6587, 9.683) knots 0 0 0 1 1 1
  spline S161 degree 2 poles (44.6587, 9.683) (44.9884, 10.0577) (45.553, 10.0577) knots 0 0 0 1 1 1
  line L149 (45.553, 10.0577) -> (47.0467, 10.0577)
  spline S162 degree 2 poles (47.0467, 10.0577) (47.3465, 10.0577) (47.3465, 9.7579) knots 0 0 0 1 1 1
  line L150 (47.3465, 9.7579) -> (47.3465, 6.1709)
  spline S163 degree 2 poles (47.3465, 6.1709) (47.3465, 5.8712) (47.0467, 5.8712) knots 0 0 0 1 1 1
  spline S164 degree 2 poles (47.0467, 5.8712) (46.747, 5.8712) (46.747, 6.1709) knots 0 0 0 1 1 1
  line L151 (46.747, 6.1709) -> (46.747, 7.6647)
  line L152 (46.747, 7.6647) -> (46.0126, 7.6647)
  line L153 (46.747, 8.2642) -> (46.747, 9.4582)
  line L154 (46.747, 9.4582) -> (45.553, 9.4582)
  spline S165 degree 2 poles (45.553, 9.4582) (45.2732, 9.4582) (44.9585, 9.1085) (44.9585, 8.8637) knots 0 0 0 1 2 2 2
  spline S166 degree 2 poles (44.9585, 8.8637) (44.9585, 8.6189) (45.1083, 8.449) knots 0 0 0 1 1 1
  spline S167 degree 2 poles (45.1083, 8.449) (45.2732, 8.2642) (45.553, 8.2642) knots 0 0 0 1 1 1
  line L155 (45.553, 8.2642) -> (46.747, 8.2642)
  point P0 (32.5, 0)
  constraints: 2 other
extrude "Выдавливание4" cut sketch "Эскиз4" against normal blind 1
